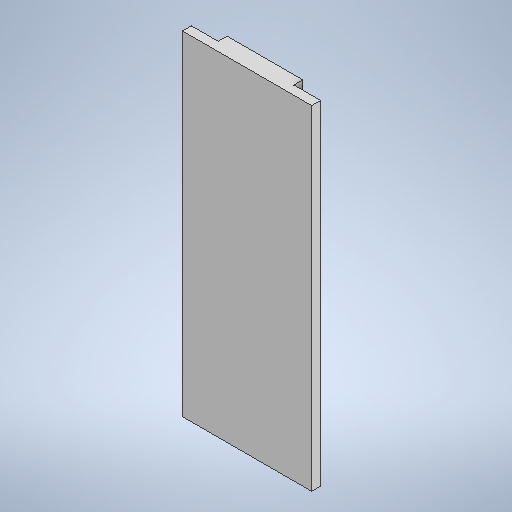
# Autodesk Inventor part: Part2
Saved by Autodesk Inventor 2025.3 (Build 293356000, 356)
## iProperties
Created: 2025-06-06
Part Number: Part2
Material: Generic
Document SubType Name: Modeling
Designer: Repete
Density: 1 g/cm^3
Appearance: Default
Author: Repete
Autodesk Inventor part; units mm, degrees
ref_plane "YZ Plane" through (0, 0, 0) normal (1, 0, 0) x (0, 1, 0)
ref_plane "XZ Plane" through (0, 0, 0) normal (0, 1, 0) x (-1, 0, 0)
ref_plane "XY Plane" through (0, 0, 0) normal (0, 0, 1) x (1, 0, 0)
sketch "Sketch1" plane through (0, 0, 0) normal (0, 1, 0) x (-1, 0, 0)
  line L0 (20.0371, 36.1085) -> (-8.9629, 36.1085)
  line L1 (-8.9629, 36.1085) -> (-8.9629, -38.8915)
  line L2 (-8.9629, -38.8915) -> (20.0371, -38.8915)
  line L3 (20.0371, -38.8915) -> (20.0371, 36.1085)
  point P0 (0, 0)
  dimension "d0" = 75
  dimension "d1" = 29
  constraints: 8 end point, 2 parallel, 1 horizontal, 1 perpendicular
  measures "d0" distance of L2.end L0.start
  measures "d1" distance of L1.end L2.end
extrude "Extrusion1" add sketch "Sketch1" along normal blind 2
sketch "Sketch2" plane through (0, 2, 0) normal (0, 1, 0) x (1, 0, 0)
  line L0 (-20.0371, -36.1085) -> (8.9629, -36.1085) projected
  line L1 (2.9629, -36.1085) -> (2.9629, 38.8915)
  line L2 (8.9629, 38.8915) -> (-20.0371, 38.8915) projected
  line L3 (-14.0371, -36.1085) -> (-14.0371, 38.8915)
  point P0 (0, 0)
  dimension "d4" = 6
  dimension "d5" = 6
  constraints: 4 end point, 2 point on line, 2 vertical
  measures "d4" distance of L3.start L0.start
  measures "d5" distance of L0.end L1.start
extrude "Extrusion2" add sketch "Sketch2" along normal blind 2
body "Solid1"
